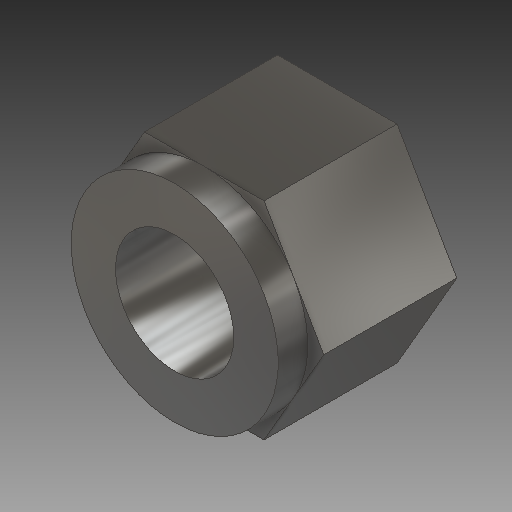
# Autodesk Inventor part: ナイロンナットm4
Saved by Autodesk Inventor 2020 (Build 240168000, 168)
## iProperties
Created: 2018-11-28
Part Number: ナイロンナットm4
Material: 鋼、高強度、低合金
Document SubType Name: Modeling
Designer: 雪村
Mass: 1.25858 g
Surface Area: 2.59963 cm^2
Volume: 0.160328 cm^3
Density: 7.85 g/cm^3
Appearance: 鋼 - つや出し
Author: 雪村
Autodesk Inventor part; units mm, degrees
ref_plane "YZ Plane" through (0, 0, 0) normal (1, 0, 0) x (0, 1, 0)
ref_plane "XZ Plane" through (0, 0, 0) normal (0, 1, 0) x (-1, 0, 0)
ref_plane "XY Plane" through (0, 0, 0) normal (0, 0, 1) x (1, 0, 0)
sketch "スケッチ1" plane through (0, 0, 0) normal (0, 0, 1) x (1, 0, 0)
  line L0 (-2.0207, 3.5) -> (2.0207, 3.5)
  line L1 (2.0207, 3.5) -> (4.0415, 0)
  line L2 (4.0415, 0) -> (2.0207, -3.5)
  line L3 (2.0207, -3.5) -> (-2.0207, -3.5)
  line L4 (-2.0207, -3.5) -> (-4.0415, 0)
  line L5 (-4.0415, 0) -> (-2.0207, 3.5)
  circle A0 centre (0, 0) radius 2
  dimension "d0" = 7
  dimension "d1" = 4
  constraints: 12 end point, 2 coincident, 1 centre point, 1 horizontal, 13 other
  measures "d0" distance between parallel lines of L3 L0
  measures "d1" diameter of A0
extrude "押し出し1" add sketch "スケッチ1" along normal blind 5.5
sketch "スケッチ2" plane through (0, 0, 5.5) normal (0, 0, 1) x (1, 0, 0)
  line L0 (2.0207, 3.5) -> (-2.0207, 3.5) projected
  line L1 (-2.0207, 3.5) -> (-4.0415, 0) projected
  line L2 (-4.0415, 0) -> (-2.0207, -3.5) projected
  line L3 (-2.0207, -3.5) -> (2.0207, -3.5) projected
  line L4 (2.0207, -3.5) -> (4.0415, 0) projected
  line L5 (4.0415, 0) -> (2.0207, 3.5) projected
  circle A0 centre (0, 0) radius 3.5
  constraints: 1 centre point, 1 coincident, 1 tangent
extrude "押し出し2" cut sketch "スケッチ2" against normal blind 1 contours L5 A0 L0 | A0 L1 L0 | L5 L4 A0 | A0 L2 L1 | A0 L3 L2 | L4 L3 A0
